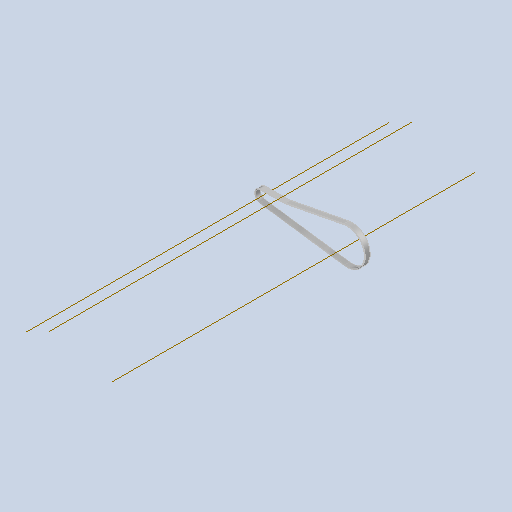
# Autodesk Inventor part: Synchronous Belt
Saved by Autodesk Inventor 2023 (Build 270158000, 158)
## iProperties
CustomPartVersion: 1
Created: 2022-01-10
Part Number: Synchronous Belt
Material: Rubber
Document SubType Name: Modeling
Designer: Jochen
Density: 1 g/cm^3
Appearance: Rubber - Black - Version 1.1
Author: Jochen
Autodesk Inventor part; units mm, degrees
sketch "Sketch Path" plane through (0, 0, 0) normal (0, 0, 1) x (1, 0, 0)
  arc A0 (9.936, -4.607) -> (9.3224, -14.1105) centre (9.981, -9.3815) ccw
  arc A1 (28.5872, -4.4313) -> (29.4465, -4.3455) centre (28.542, 0.3685) ccw
  arc A2 (77.2347, -23.5685) -> (76.5111, 4.6858) centre (79.2105, -9.3815) ccw
  line L0 (77.2347, -23.5685) -> (9.3224, -14.1105)
  line L1 (9.936, -4.607) -> (28.5872, -4.4313)
  line L2 (29.4465, -4.3455) -> (76.5111, 4.6858)
  constraints: 6 end point, 6 point on circle, 3 centre point
ref_plane "Cross Section Plane" through (9.3224, -14.1105, 0) normal (0.9904, -0.1379, 0) x (0, 0, 1)
ref_plane "Work Plane2" through (9.981, -9.3815, 0) normal (-1, 0, 0) x (0, 0, 1)
ref_plane "Work Plane3" through (79.2105, -9.3815, 0) normal (-0.9998, -0.0189, 0) x (0, 0, 1)
sketch "Cross Section" plane through (9.3224, -14.1105, 0) normal (0.9904, -0.1379, 0) x (0, 0, 1)
  line L0 (-2, 0.3) -> (2, 0.3)
  line L1 (2, 0.3) -> (2, -0.3)
  line L2 (2, -0.3) -> (-2, -0.3)
  line L3 (-2, -0.3) -> (-2, 0.3)
  line L4 (-2, 0) -> (2, 0) construction
  point P0 (0, 0)
  point P1 (0, 0)
  dimension "d0" = 4
  dimension "d4" = 0.3
  dimension "d5" = 0.3
  constraints: 10 end point, 3 midpoint, 2 parallel, 1 coincident, 1 horizontal, 1 perpendicular, 1 other
  measures "d0" distance between parallel lines of L1 L3
  measures "d4" distance between parallel lines of L2 L4
  measures "d5" distance between parallel lines of L4 L0
sweep "Belt" add profiles "Cross Section" path "Sketch Path"
equation "\"d0\" = da_B"
equation "\"d4\" = da_a"
equation "\"d5\" = da_a2"
equation "\"da_B\" = 4"
equation "\"da_pb\" = 2.5"
equation "\"da_a\" = 0.3"
equation "\"da_S\" = 1.5"
equation "\"da_Beta\" = 20deg"
equation "\"da_Ht\" = 0.7"
equation "\"da_H\" = 1.3"
equation "\"da_a2\" = 0.3"
body "Solid1"
